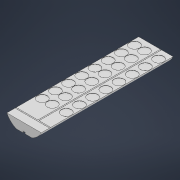
# Autodesk Inventor part: Floor
Saved by Autodesk Inventor 2021 (Build 250183000, 183)
## iProperties
Created: 2021-01-31
Part Number: Floor
Material: Generic
Document SubType Name: Modeling
Designer: argon
Density: 1 g/cm^3
Appearance: Light Gray
Author: argon
Autodesk Inventor part; units mm, degrees
ref_plane "YZ Plane" through (0, 0, 0) normal (1, 0, 0) x (0, 1, 0)
ref_plane "XZ Plane" through (0, 0, 0) normal (0, 1, 0) x (-1, 0, 0)
ref_plane "XY Plane" through (0, 0, 0) normal (0, 0, 1) x (1, 0, 0)
sketch "Sketch1" plane through (0, 0, 0) normal (0, 0, 1) x (1, 0, 0)
  circle A0 centre (0, 0) radius 1750
  line L0 (-1569.0363, -775) -> (1569.0363, -775)
  line L1 (-64, -1498) -> (64, -1498)
  line L2 (64, -1498) -> (64, -1600)
  line L3 (64, -1600) -> (-64, -1600)
  line L4 (-64, -1600) -> (-64, -1498)
  line L5 (-64, -1498) -> (64, -1600) construction
  line L6 (64, -1498) -> (-64, -1600) construction
  line L7 (97, -1633) -> (97, -1465)
  line L8 (97, -1465) -> (-97, -1465)
  line L9 (-97, -1465) -> (-97, -1633)
  line L10 (-97, -1633) -> (97, -1465) construction
  line L11 (97, -1633) -> (-97, -1465) construction
  line L12 (-708.8723, -1600) -> (708.8723, -1600)
  point P0 (0, -1549)
  point P1 (0, -1549)
  point P2 (97, -1600)
  point P3 (-97, -1600)
  dimension "d10" = 3500
  dimension "d12" = 33
  dimension "d13" = 33
  dimension "d14" = 102
  dimension "d15" = 128
  dimension "d16" = 1600
  dimension "d17" = 825
  constraints: 26 end point, 5 midpoint, 4 point on circle, 3 horizontal, 3 parallel, 1 centre point, 1 coincident, 1 collinear, 1 perpendicular, 1 vertical alignment
  measures "d10" diameter of A0
  measures "d12" distance between parallel lines of L2 L7
  measures "d13" distance between parallel lines of L1 L8
  measures "d14" distance of L2.start L2.end
  measures "d15" distance of L4.end L2.start
  measures "d16" distance from line of L3 point (0, 0)
  measures "d17" distance between parallel lines of L12 L0
extrude "Extrusion1" add sketch "Sketch1" along normal blind 12000 contours L0 A0 L12 L7 L8 L9
sketch "Sketch2" plane through (-1569.0363, -775, 0) normal (0, 1, 0) x (1, 0, 0)
  circle A0 centre (2663.0727, -9252.935) radius 450
  circle A1 centre (1385, -9252.935) radius 450
  circle A2 centre (475, -9252.935) radius 450
  line L0 (3138.0727, 0) -> (3138.0727, -12000) projected
  line L1 (0, 0) -> (0, -12000) projected
  circle A3 centre (475, -8052.935) radius 450
  circle A4 centre (1385, -8052.935) radius 450
  circle A5 centre (2663.0727, -8052.935) radius 450
  circle A6 centre (475, -6852.935) radius 450
  circle A7 centre (1385, -6852.935) radius 450
  circle A8 centre (2663.0727, -6852.935) radius 450
  circle A9 centre (475, -5652.935) radius 450
  circle A10 centre (1385, -5652.935) radius 450
  circle A11 centre (2663.0727, -5652.935) radius 450
  circle A12 centre (475, -4452.935) radius 450
  circle A13 centre (1385, -4452.935) radius 450
  circle A14 centre (2663.0727, -4452.935) radius 450
  circle A15 centre (475, -3252.935) radius 450
  circle A16 centre (1385, -3252.935) radius 450
  circle A17 centre (2663.0727, -3252.935) radius 450
  circle A18 centre (475, -2052.935) radius 450
  circle A19 centre (1385, -2052.935) radius 450
  circle A20 centre (2663.0727, -2052.935) radius 450
  circle A21 centre (475, -852.935) radius 450
  circle A22 centre (1385, -852.935) radius 450
  circle A23 centre (2663.0727, -852.935) radius 450
  point P0 (1569.0363, 0)
  dimension "d20" = 900
  dimension "d21" = 910
  dimension "d24" = 1200
  dimension "d31" = 475
  dimension "d32" = 475
  constraints: 24 centre point, 2 equal radius, 2 horizontal alignment, 1 vertical, 42 other
  measures "d20" diameter of A2
  measures "d21" distance of A1.centre A2.centre
  measures "d24" distance of A2.centre A3.centre
  measures "d31" distance from line of L1 A2.centre
  measures "d32" distance from line of L0 A0.centre
extrude "Extrusion2" cut sketch "Sketch2" against normal blind 20
sketch "Sketch3" plane through (-1569.0363, -775, 0) normal (0, 1, 0) x (1, 0, 0)
  line L0 (1666.0363, 0) -> (2277.9087, 0) projected
  line L1 (2074.0363, 0) -> (1974.0363, 0)
  line L2 (1974.0363, 0) -> (1974.0363, -11147.7438)
  line L3 (1974.0363, -11147.7438) -> (2074.0363, -11147.7438)
  line L4 (2074.0363, -11147.7438) -> (2074.0363, 0)
  line L5 (0, 0) -> (0, -12000) projected
  line L6 (3138.0727, -11247.7438) -> (0, -11247.7438)
  line L7 (0, -11247.7438) -> (0, -11147.7438)
  line L8 (0, -11147.7438) -> (3138.0727, -11147.7438)
  line L9 (3138.0727, -11147.7438) -> (3138.0727, -11247.7438)
  line L10 (3138.0727, 0) -> (3138.0727, -12000) projected
  circle A0 centre (2663.0727, -9252.935) radius 450 projected
  circle A1 centre (2024.0363, -9581.3845) radius 268.503 construction
  circle A2 centre (1385, -9252.935) radius 450 projected
  line L11 (2024.0363, -9581.3845) -> (1974.0363, -9581.3845) construction
  line L12 (2024.0363, -9581.3845) -> (2074.0363, -9581.3845) construction
  point P0 (1569.0363, 0)
  dimension "d33" = 100
  constraints: 20 end point, 5 point on line, 4 parallel, 4 perpendicular, 2 equal length, 2 horizontal, 2 tangent, 1 centre point, 1 collinear
  measures "d33" distance between parallel lines of L2 L4
extrude "Extrusion3" cut sketch "Sketch3" against normal blind 5 contours L0 L4 L3 L2 | L3 L8 L9 L6 L5
body "Solid1"
